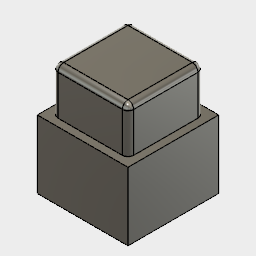
Nibbler - Button Extension (Autodesk Fusion 360 design; units mm, degrees)
Autodesk Fusion 360 part; units mm, degrees
sketch "Sketch1" plane through (0, 0, 0) normal (0, 1, 0) x (1, 0, 0)
  line L0 (0, 0) -> (12, 0)
  line L1 (12, 0) -> (12, 12)
  line L2 (12, 12) -> (0, 12)
  line L3 (0, 12) -> (0, 0)
  dimension "d1" = 12
  dimension "d2" = 12
  constraint horizontal L0
  constraint vertical L1
  constraint horizontal L2
  constraint vertical L3
  constraint coincident L0.start L3.end
extrude "Extrude1" add sketch "Sketch1" along normal blind 9
sketch "Sketch2" plane through (0, 9, 0) normal (0, 1, 0) x (-1, 0, 0)
  line L0 (0, -12) -> (0, 0)
  line L1 (0, 0) -> (-12, 0)
  line L2 (-12, 0) -> (-12, -12)
  line L3 (-12, -12) -> (0, -12)
  line L4 (-11, -1) -> (-1, -1)
  line L5 (-1, -1) -> (-1, -11)
  line L6 (-1, -11) -> (-11, -11)
  line L7 (-11, -11) -> (-11, -1)
  line L8 (-11, -1) -> (-1, -11) construction
  line L9 (-1, -1) -> (-11, -11) construction
  dimension "d5" = 10
  dimension "d6" = 10
  constraint perpendicular L4 L5
  constraint parallel L4 L6
  constraint parallel L5 L7
  constraint horizontal L4
  constraint coincident L8 L0.end
  constraint coincident L9 L0.end
extrude "Extrude2" add sketch "Sketch2" along normal blind 6 contours L4 L5 L6 L7
fillet "Fillet1" radius 0.75 8 edges at (1, 12, -1) (11, 12, -1) (6, 15, -1) (11, 15, -6) (6, 15, -11) (1, 15, -6) (11, 12, -11) (1, 12, -11)
sketch "Sketch5" plane through (0, 0, 0) normal (0, -1, 0) x (1, 0, 0)
  line L0 (0, 0) -> (0, -12)
  line L1 (0, -12) -> (12, -12)
  line L2 (12, -12) -> (12, 0)
  line L3 (12, 0) -> (0, 0)
  line L4 (8.2, -8.2) -> (3.8, -8.2)
  line L5 (3.8, -8.2) -> (3.8, -3.8)
  line L6 (3.8, -3.8) -> (8.2, -3.8)
  line L7 (8.2, -3.8) -> (8.2, -8.2)
  line L8 (8.2, -8.2) -> (3.8, -3.8) construction
  line L9 (3.8, -8.2) -> (8.2, -3.8) construction
  line L10 (8.1, -8.1) -> (3.9, -8.1)
  line L11 (3.9, -8.1) -> (3.9, -3.9)
  line L12 (3.9, -3.9) -> (8.1, -3.9)
  line L13 (8.1, -3.9) -> (8.1, -8.1)
  line L14 (8.1, -8.1) -> (3.9, -3.9) construction
  line L15 (3.9, -8.1) -> (8.1, -3.9) construction
  dimension "d24" = 4.4
  dimension "d25" = 4.4
  dimension "d28" = 4.2
  dimension "d29" = 4.2
  constraint perpendicular L4 L5
  constraint parallel L4 L6
  constraint parallel L5 L7
  constraint horizontal L4
  constraint coincident L8 L0.start
  constraint coincident L9 L0.start
  constraint perpendicular L10 L11
  constraint parallel L10 L12
  constraint parallel L11 L13
  constraint horizontal L10
  constraint coincident L14 L0.start
  constraint coincident L15 L0.start
  constraint coincident L0.start L3.end
extrude "Extrude6" cut sketch "Sketch5" against normal blind 7 contours L4 L5 L6 L7 | L10 L11 L12 L13
extrude "Extrude7" add sketch "Sketch5" against normal blind 1.5 contours L4 L5 L6 L7
chamfer "Chamfer3" distance 1.5 angle 45 4 edges at (3.8, 7, -6) (6, 7, -8.2) (6, 7, -3.8) (8.2, 7, -6)
named bodies: "Button Extension"
